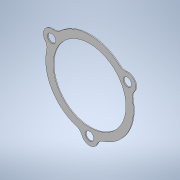
# Autodesk Inventor part: 79. Прокладка
Saved by Autodesk Inventor 2021 (Build 250183000, 183)
## iProperties
Created: 2021-03-15
Part Number: 79. Прокладка
Material: Типовые
Document SubType Name: Modeling
Designer: Данил
Density: 1 g/cm^3
Appearance: По умолчанию
Author: Данил
Autodesk Inventor part; units mm, degrees
ref_plane "YZ Plane" through (0, 0, 0) normal (1, 0, 0) x (0, 1, 0)
ref_plane "XZ Plane" through (0, 0, 0) normal (0, 1, 0) x (-1, 0, 0)
ref_plane "XY Plane" through (0, 0, 0) normal (0, 0, 1) x (1, 0, 0)
sketch "Эскиз1" plane through (0, 0, 0) normal (0, 0, 1) x (1, 0, 0)
  circle A0 centre (0, 0) radius 44
  circle A1 centre (-45.8993, 26.5) radius 5
  circle A2 centre (45.8993, 26.5) radius 5
  circle A3 centre (0, -53) radius 5
  line L0 (0, 0) -> (-45.8993, 26.5) construction
  line L1 (0, 0) -> (45.8993, 26.5) construction
  line L2 (0, -53) -> (0, 0) construction
  arc A4 (-51.6909, 11.7068) -> (-53.6716, 20.2078) centre (-61.4439, 13.9156) ccw
  arc A5 (-44.3363, 36.3771) -> (-53.6716, 20.2078) centre (-45.8993, 26.5) ccw
  arc A6 (-44.3363, 36.3771) -> (-35.9838, 38.9122) centre (-42.7733, 46.2542) ccw
  arc A7 (35.9838, 38.9122) -> (44.3363, 36.3771) centre (42.7733, 46.2542) ccw
  arc A8 (53.6716, 20.2078) -> (44.3363, 36.3771) centre (45.8993, 26.5) ccw
  arc A9 (53.6716, 20.2078) -> (51.6909, 11.7068) centre (61.4439, 13.9156) ccw
  arc A10 (15.7071, -50.619) -> (9.3353, -56.5849) centre (18.6707, -60.1698) ccw
  arc A11 (-9.3353, -56.5849) -> (9.3353, -56.5849) centre (0, -53) ccw
  arc A12 (-9.3353, -56.5849) -> (-15.7071, -50.619) centre (-18.6707, -60.1698) ccw
  arc A13 (4.9944, -52.7642) -> (0, -53) centre (0, 0) ccw construction
  arc A14 (35.9838, 38.9122) -> (-35.9838, 38.9122) centre (0, 0) ccw
  arc A15 (-51.6909, 11.7068) -> (-15.7071, -50.619) centre (0, 0) ccw
  arc A16 (15.7071, -50.619) -> (51.6909, 11.7068) centre (0, 0) ccw
  dimension "d0" = 88
  dimension "d2" = 10
  dimension "d3" = 120
  dimension "d4" = 120
  dimension "d6" = 10
  dimension "d7" = 106
  dimension "d8" = 53
  dimension "d10" = 53
  constraints: 28 point on circle, 16 centre point, 13 tangent, 9 equal radius, 6 coincident, 6 end point, 1 vertical, 4 other
  measures "d0" diameter of A0
  measures "d2" diameter of A1
  measures "d3" angle of L0 L1
  measures "d4" angle of L2 L0
  measures "d6" radius of A5
  measures "d7" diameter of A13
  measures "d8" radius of A14
  measures "d10" radius of A15
extrude "Выдавливание1" add sketch "Эскиз1" along normal mid plane 1
